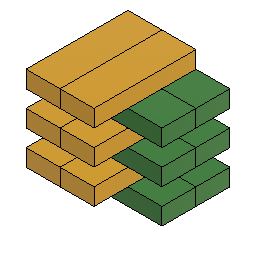
08-TopLevelComponentsAsOneFile (Autodesk Fusion 360 design; units mm, degrees)
Autodesk Fusion 360 part; units mm, degrees
sketch "Sketch1" plane through (0, 0, 0) normal (0, 0, 1) x (1, 0, 0)
  line L0 (30, -10) -> (-30, -10)
  line L1 (-30, -10) -> (-30, 10)
  line L2 (-30, 10) -> (30, 10)
  line L3 (30, 10) -> (30, -10)
  line L4 (30, -10) -> (-30, 10) construction
  line L5 (-30, -10) -> (30, 10) construction
  dimension "length" = 60
  dimension "width" = 20
  constraint horizontal L0
  constraint perpendicular L0 L1
  constraint parallel L0 L2
  constraint parallel L1 L3
  constraint coincident L4 origin
  constraint coincident L5 origin
  measures "length" distance of L1.end L2.end
  measures "width" distance of L0.end L1.end
extrude "Extrude1" add sketch "Sketch1" along normal blind 10 makes body 1 in component "green"
pattern_linear "R-Pattern1" count 3 spacing 20 along (0, 0, 1) of bodies 1 makes body 2 at (10, -3.3333, 20) makes body 3 at (10, -3.3333, 40) in component "green"
extrude "Extrude1'" add sketch "Sketch1" along normal blind 10 from surface at 10 separate body makes body 4 in component "block"
pattern_linear "ᜁ3" [suppressed] in component "yellow"
pattern_linear "焁4" [suppressed] in component "red"
pattern_linear "" [suppressed]
component "green" placed x (1, 0, 0) y (0, 1, 0) z (0, 0, 1) at (0, 0, 0)
component "yellow" placed x (1, 0, 0) y (0, 1, 0) z (0, 0, 1) at (0, 0, 0)
component "red" placed x (1, 0, 0) y (0, 1, 0) z (0, 0, 1) at (0, 0, 0)
component "green" placed x (1, 0, 0) y (0, 1, 0) z (0, 0, 1) at (0, 20, 0)
component "block" placed x (0, -1, 0) y (1, 0, 0) z (0, 0, 1) at (0, 0, 0) in component "yellow"
component "block" placed x (0, -1, 0) y (1, 0, 0) z (0, 0, 1) at (0, 0, 20) in component "yellow"
component "block" placed x (0, -1, 0) y (1, 0, 0) z (0, 0, 1) at (0, 0, 40) in component "yellow"
component "block" placed x (0, -1, 0) y (1, 0, 0) z (0, 0, 1) at (-20, 0, 0) in component "red"
component "block" placed x (0, -1, 0) y (1, 0, 0) z (0, 0, 1) at (-20, 0, 20) in component "red"
component "block" placed x (0, -1, 0) y (1, 0, 0) z (0, 0, 1) at (-20, 0, 40) in component "red"
equation "height = 10 mm"
equation "d4 = height"
equation "d8 = height * 2"
equation "d14 = height"
equation "d18 = height * 2"
equation "d22 = height * 2"
equation "d26 = width"
named bodies: "greenBlock1", "greenBlock1 (1)", "greenBlock1 (2)"
